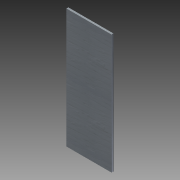
# Autodesk Inventor part: Part12
Saved by Autodesk Inventor 2011 SP1 (Build 150282100, 282)
## iProperties
Created: 2011-06-11
Part Number: Part12
Document SubType Name: Modeling
Designer: Andrew G. Meyer
Mass: 46.2601 g
Surface Area: 310.841 cm^2
Volume: 46.2601 cm^3
Density: 1 g/cm^3
Author: Andrew G. Meyer
Autodesk Inventor part; units mm, degrees
ref_plane "YZ Plane" through (0, 0, 0) normal (1, 0, 0) x (0, 1, 0)
ref_plane "XZ Plane" through (0, 0, 0) normal (0, 1, 0) x (-1, 0, 0)
ref_plane "XY Plane" through (0, 0, 0) normal (0, 0, 1) x (1, 0, 0)
sketch "Sketch1" plane through (0, 0, 0) normal (0, 0, 1) x (1, 0, 0)
  line L0 (-19.651, 120.0641) -> (56.549, 120.0641)
  line L1 (56.549, 120.0641) -> (56.549, -76.7859)
  line L2 (56.549, -76.7859) -> (-19.651, -76.7859)
  line L3 (-19.651, -76.7859) -> (-19.651, 120.0641)
  point P0 (0, 0)
  dimension "d0" = 196.85
  dimension "d1" = 76.2
  constraints: 8 end point, 2 parallel, 1 horizontal, 1 perpendicular
  measures "d0" distance of L0.end L1.end
  measures "d1" distance of L1.end L2.end
extrude "Extrusion1" add sketch "Sketch1" along normal blind 3.175
hole "Hole1" at (56.549, 120.0641, 1.5875) direction (0, -1, 0) diameter 4.7498 depth 228.6 tip angle 118
body "Solid1"
